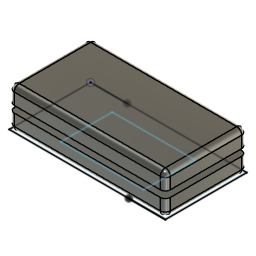
wilson jawn v1 (Autodesk Fusion 360 design; units mm, degrees)
Autodesk Fusion 360 part; units mm, degrees
sketch "Sketch1" plane through (0, 0, 0) normal (0, 0, 1) x (1, 0, 0)
  line L0 (0, 0) -> (23.5, 0)
  line L1 (0, 0) -> (0, -12.25)
  line L2 (0, -12.25) -> (23.5, -12.25)
  line L3 (23.5, 0) -> (23.5, -12.25)
  line L4 (0, 0) -> (5.5, 0)
  line L5 (23.5, -12.25) -> (18, -12.25)
  line L6 (18, -10) -> (5.5, -10)
  line L7 (5.5, -10) -> (5.5, -2.25)
  line L8 (5.5, -2.25) -> (18, -2.25)
  line L9 (18, -2.25) -> (18, -10)
  dimension "d1" = 23.5
  dimension "d2" = 12.25
  dimension "d3" = 5.5
  dimension "d4" = 2.25
  dimension "d5" = 5.5
  dimension "d6" = 2.25
  constraint coincident L0.start L1.start
  constraint horizontal L0
  constraint perpendicular L0 L1
  constraint perpendicular L1 L2
  constraint perpendicular L2 L3
  constraint perpendicular L1 L4
  constraint perpendicular L3 L5
  constraint horizontal L6
  constraint vertical L7
  constraint horizontal L8
  constraint vertical L9
  measures "d1" distance of L0.start L0.end
  measures "d2" distance of L0.start L1.end
  measures "d3" distance of L0.start L4.end
  measures "d4" distance of L4.end L7.end
  measures "d5" distance of L2.end L5.end
  measures "d6" distance of L5.end L6.start
extrude "Extrude1" add sketch "Sketch1" along normal blind 6 contours L6 L7 L8 L9 makes body 1
extrude "Extrude2" add sketch "Sketch1" along normal blind 6 separate body makes body 2
sketch "Sketch2" plane through (23.5, 0, 0) normal (1, 0, 0) x (0, 1, 0)
  line L0 (-12.25, 0) -> (0, 0)
  line L1 (0, 0) -> (0, 6)
  line L2 (0, 6) -> (-12.25, 6)
  line L3 (-12.25, 6) -> (-12.25, 0)
  line L4 (0, 3.5) -> (-2.25, 3.5)
  line L5 (-12.25, 2.5) -> (-10, 2.5)
  line L6 (-12.25, 2.5) -> (0, 2.5)
  line L7 (0, 2.5) -> (0, 3.5)
  line L8 (0, 3.5) -> (-12.25, 3.5)
  line L9 (-12.25, 3.5) -> (-12.25, 2.5)
  dimension "d12" = 2.25
  dimension "d13" = 2.5
  dimension "d14" = 2.25
  constraint coincident L1 L4.start
  constraint perpendicular L1 L4
  constraint horizontal L6
  constraint vertical L7
  constraint horizontal L8
  constraint vertical L9
  measures "d12" distance of L4.start L4.end
  measures "d13" distance of L0.start L5.start
  measures "d14" distance of L5.start L5.end
extrude "Extrude3" cut sketch "Sketch2" against normal blind 29 contours L1 L3 L4 L5 L6 L7 L8 L9 bodies 1 2 makes body 4 at (1.8333, -4.8333, 3.5) makes body 3 at (9.6667, -4.8333, 3.5)
extrude "Extrude4" add 1 faces at (13.8333, -7.4167, 2.5) along direction (0, 0, 1) blind 2 on bodies 1 bodies 1 2 3 4
fillet "Fillet1" radius 0.75 16 edges at (0, 0, 4.75) (11.75, 0, 6) (0, -6.125, 6) (11.75, -12.25, 6) (0, -12.25, 4.75) (23.5, -12.25, 4.75) (23.5, -6.125, 6) (23.5, 0, 4.75) (11.75, 0, 0) (0, 0, 1.25) (0, -6.125, 0) (0, -12.25, 1.25) (11.75, -12.25, 0) (23.5, -12.25, 1.25) (23.5, -6.125, 0) (23.5, 0, 1.25) on bodies 1
